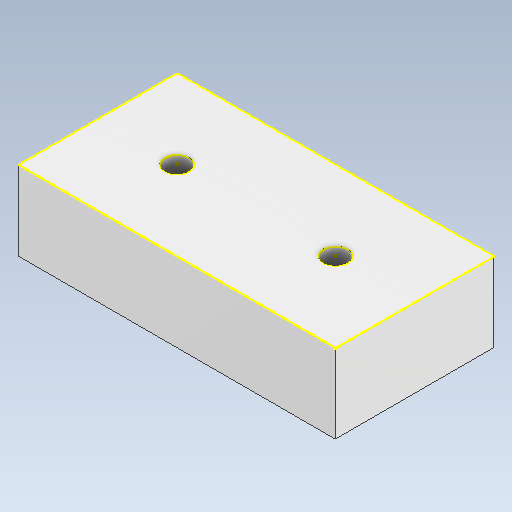
# Autodesk Inventor part: front delrin
Saved by Autodesk Inventor 2020.1 (Build 241239000, 239)
## iProperties
Created: 2019-11-10
Part Number: front delrin
Material: UHMW, White
Document SubType Name: Modeling
Designer: amirs
Density: 0.94 g/cm^3
Appearance: Smooth - White
Mass: 1.89054 g
Surface Area: 11.9434 cm^2
Volume: 2.01121 cm^3
Author: amirs
Autodesk Inventor part; units mm, degrees
ref_plane "YZ Plane" through (0, 0, 0) normal (1, 0, 0) x (0, 1, 0)
ref_plane "XZ Plane" through (0, 0, 0) normal (0, 1, 0) x (-1, 0, 0)
ref_plane "XY Plane" through (0, 0, 0) normal (0, 0, 1) x (1, 0, 0)
sketch "Sketch1" plane through (0, 0, 0) normal (0, 1, 0) x (-1, 0, 0)
  line L0 (0, 0) -> (25.4, 0)
  line L1 (25.4, 0) -> (25.4, -12.7)
  line L2 (25.4, -12.7) -> (0, -12.7)
  line L3 (0, -12.7) -> (0, 0)
  line L4 (25.4, -6.35) -> (0, -6.35) construction
  circle A0 centre (19.05, -6.35) radius 0.9652
  circle A1 centre (6.35, -6.35) radius 0.9652
  dimension "d0" = 12.7
  dimension "d1" = 25.4
  dimension "d2" = 1.9304
  dimension "d3" = 12.7
  dimension "d4" = 6.35
  constraints: 10 end point, 2 centre point, 2 midpoint, 2 parallel, 2 point on line, 1 equal radius, 1 horizontal, 1 perpendicular
  measures "d0" distance of L2.end L0.start
  measures "d1" distance of L1.end L2.end
  measures "d2" diameter of A0
  measures "d3" distance of A1.centre A0.centre
  measures "d4" distance from line of L1 A0.centre
extrude "Extrusion1" add sketch "Sketch1" along normal blind 6.35
sketch "Sketch2" plane through (0, 6.35, 0) normal (0, 1, 0) x (1, 0, 0)
  line L0 (0, 12.7) -> (-25.4, 12.7) projected
  line L1 (-25.4, 12.7) -> (-25.4, 0) projected
  line L2 (-25.4, 0) -> (0, 0) projected
  line L3 (0, 0) -> (0, 12.7) projected
  circle A0 centre (-6.35, 6.35) radius 0.9652 projected
  circle A1 centre (-19.05, 6.35) radius 0.9652 projected
body "Solid1"
